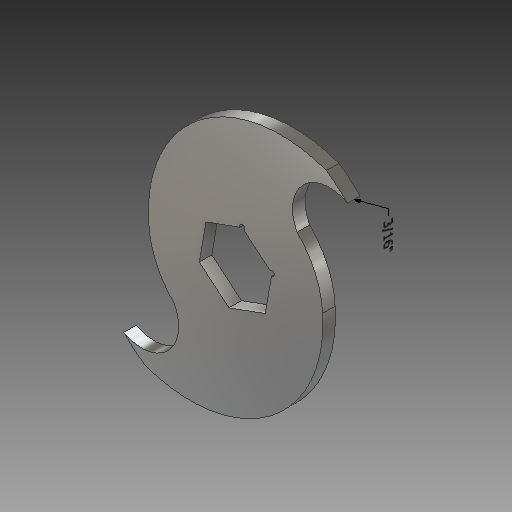
# Autodesk Inventor part: 3-16inch_Knife2_Piece1
Saved by Autodesk Inventor 2018 (Build 220112000, 112)
## iProperties
Created: 2018-01-21
Part Number: 3-16inch_Knife2_Piece1
Material: Generic
Document SubType Name: Modeling
Designer: Olivier
Density: 1 g/cm^3
Appearance: Default
Mass: 22.6509 g
Surface Area: 115.828 cm^2
Volume: 22.6509 cm^3
Author: Olivier
Autodesk Inventor part; units mm, degrees
ref_plane "YZ Plane" through (0, 0, 0) normal (1, 0, 0) x (0, 1, 0)
ref_plane "XZ Plane" through (0, 0, 0) normal (0, 1, 0) x (-1, 0, 0)
ref_plane "XY Plane" through (0, 0, 0) normal (0, 0, 1) x (1, 0, 0)
sketch "Sketch1" plane through (0, 0, 0) normal (0, 0, 1) x (1, 0, 0)
  arc A0 (-117.4264, -42.4264) -> (-98.3345, -23.3345) centre (-110.6099, -30.151) ccw
  arc A1 (-117.4264, -42.4264) -> (-109.4264, -49.1408) centre (-75, 0) ccw
  arc A2 (-109.4264, -49.1408) -> (-42.0349, 1.5164) centre (-92.1264, -2.0002) ccw
  arc A3 (-42.0349, 1.5164) -> (-51.6655, 23.3345) centre (-75, 0) ccw
  arc A4 (-32.5736, 42.4264) -> (-51.6655, 23.3345) centre (-39.3901, 30.151) ccw
  arc A5 (-32.5736, 42.4264) -> (-40.5736, 49.1408) centre (-75, 0) ccw
  arc A6 (-40.5736, 49.1408) -> (-107.9651, -1.5164) centre (-57.8736, 2.0002) ccw
  arc A7 (-107.9651, -1.5164) -> (-98.3345, -23.3345) centre (-75, 0) ccw
  line L0 (-71.6875, 13.7991) -> (-61.9857, 5.6584)
  arc A8 (-61.3933, 4.0308) -> (-61.9857, 5.6584) centre (-61.2197, 5.0156) ccw
  line L1 (-61.3933, 4.0308) -> (-63.7662, -9.4263)
  line L2 (-63.7662, -9.4263) -> (-77.5465, -14.4419)
  line L3 (-77.5465, -14.4419) -> (-88.7803, -5.0156)
  line L4 (-88.7803, -5.0156) -> (-86.2338, 9.4263)
  line L5 (-86.2338, 9.4263) -> (-73.3932, 14.0999)
  arc A9 (-71.6875, 13.7991) -> (-73.3932, 14.0999) centre (-72.4535, 14.4419) ccw
  arc A10 (-109.4264, -49.1408) -> (-42.0349, 1.5164) centre (-92.1264, -2.0002) ccw
  arc A11 (-117.4264, -42.4264) -> (-109.4264, -49.1408) centre (-75, 0) ccw
  arc A12 (-117.4264, -42.4264) -> (-98.3345, -23.3345) centre (-110.6099, -30.151) ccw
  arc A13 (-107.9651, -1.5164) -> (-98.3345, -23.3345) centre (-75, 0) ccw
  arc A14 (-40.5736, 49.1408) -> (-107.9651, -1.5164) centre (-57.8736, 2.0002) ccw
  arc A15 (-32.5736, 42.4264) -> (-40.5736, 49.1408) centre (-75, 0) ccw
  arc A16 (-32.5736, 42.4264) -> (-51.6655, 23.3345) centre (-39.3901, 30.151) ccw
  arc A17 (-42.0349, 1.5164) -> (-51.6655, 23.3345) centre (-75, 0) ccw
  arc A18 (-109.4264, -49.1408) -> (-42.0349, 1.5164) centre (-92.1264, -2.0002) ccw
  point P0 (0, 0)
  constraints: 38 point on circle, 19 centre point, 12 end point
extrude "Extrusion1" add sketch "Sketch1" along normal blind 4.7625
body "Solid1"
